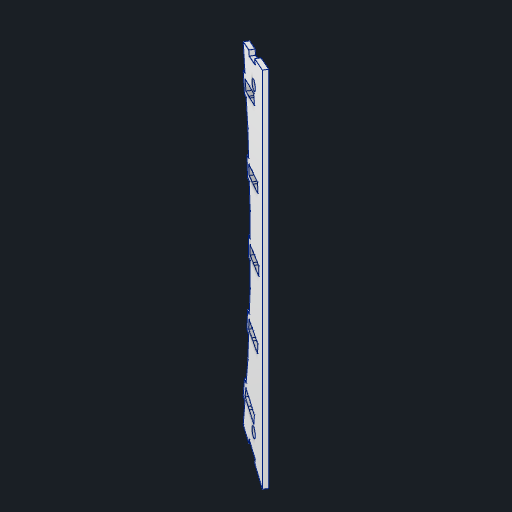
# Autodesk Inventor part: Front Plate
Saved by Autodesk Inventor 2023 (Build 270158000, 158)
## iProperties
Created: 2022-06-14
Part Number: Front Plate
Material: Aluminum 6061
Document SubType Name: Modeling
Designer: FizzyApple12
Density: 2.7 g/cm^3
Appearance: Aluminum - Flat
Author: FizzyApple12
Autodesk Inventor part; units mm, degrees
ref_plane "YZ Plane" through (0, 0, 0) normal (1, 0, 0) x (0, 1, 0)
ref_plane "XZ Plane" through (0, 0, 0) normal (0, 1, 0) x (-1, 0, 0)
ref_plane "Work Plane1" through (3.175, 0, 0) normal (0.5244795, 0, -0.8514231) x (-0.8328174, 0.2079117, -0.5130184)
sketch "Sketch1" plane through (3.175, 0, 0) normal (0.5244795, 0, -0.8514231) x (-0.8328174, 0.2079117, -0.5130184)
  line L0 (-4.273, 0.9083) -> (1.0154, -0.2158) construction
  line L1 (3.6558, 12.2067) -> (-1.6326, 13.3307) construction
  line L2 (-4.273, 0.9083) -> (-7.6513, -14.9853) projected
  line L3 (1.7457, 29.2243) -> (-1.6326, 13.3307) projected
  line L4 (6.9133, 45.2244) -> (1.8922, 29.771) projected
  line L5 (6.9133, 45.2244) -> (12.0552, 43.5536) construction
  line L6 (15.9798, 55.6321) -> (10.8378, 57.3028) construction
  line L7 (15.8589, 72.7562) -> (10.8378, 57.3028) projected
  line L8 (22.6707, 88.1284) -> (16.0618, 73.2845) projected
  line L9 (32.7754, 97.5314) -> (27.8362, 99.7304) construction
  line L10 (22.6707, 88.1284) -> (27.6098, 85.9294) construction
  line L11 (34.4452, 114.5743) -> (27.8362, 99.7304) projected
  line L12 (1.0154, -0.2158) -> (2.6442, -0.562) construction
  line L13 (2.6442, -0.562) -> (5.2847, 11.8604) construction
  line L14 (5.2847, 11.8604) -> (3.6558, 12.2067) construction
  line L15 (13.639, 43.0391) -> (17.5635, 55.1175) construction
  line L16 (12.0552, 43.5536) -> (13.639, 43.0391) construction
  line L17 (17.5635, 55.1175) -> (15.9798, 55.6321) construction
  line L18 (27.6098, 85.9294) -> (29.1311, 85.2521) construction
  line L19 (29.1311, 85.2521) -> (34.2966, 96.8541) construction
  line L20 (34.2966, 96.8541) -> (32.7754, 97.5314) construction
  line L21 (-12.4939, -90.0078) -> (-12.4939, -106.2565) projected
  line L22 (-12.4939, -90.0078) -> (-7.0873, -90.0078) construction
  line L23 (-7.0873, -90.0078) -> (-5.4221, -90.0078) construction
  line L24 (-5.4221, -90.0078) -> (-5.4221, -77.3078) construction
  line L25 (-5.4221, -77.3078) -> (-7.0873, -77.3078) construction
  line L26 (-7.0873, -77.3078) -> (-12.4939, -77.3078) construction
  line L27 (-12.4939, -61.0592) -> (-12.4939, -77.3078) projected
  line L28 (-10.7658, -44.3344) -> (-12.4643, -60.494) projected
  line L29 (-10.7658, -44.3344) -> (-5.3889, -44.8995) construction
  line L30 (-5.3889, -44.8995) -> (-3.7328, -45.0736) construction
  line L31 (-3.7328, -45.0736) -> (-2.4053, -32.4431) construction
  line L32 (-2.4053, -32.4431) -> (-4.0614, -32.2691) construction
  line L33 (-4.0614, -32.2691) -> (-9.4383, -31.7039) construction
  line L34 (-7.7398, -15.5443) -> (-9.4383, -31.7039) projected
  line L35 (-7.6513, -14.9853) -> (-7.7398, -15.5443)
  line L36 (-12.4939, -61.0592) -> (-12.4643, -60.494)
  line L37 (16.0618, 73.2845) -> (15.8589, 72.7562)
  line L38 (1.7457, 29.2243) -> (1.8922, 29.771)
  line L39 (-5.4221, -90.0078) -> (-12.4939, -90.0078)
  line L40 (-12.4939, -77.3078) -> (-5.4221, -77.3078)
  line L41 (-8.958, -90.0078) -> (-8.958, -77.3078)
  line L42 (-10.7658, -44.3344) -> (-3.7328, -45.0736)
  line L43 (-2.4053, -32.4431) -> (-9.4383, -31.7039)
  line L44 (-5.9218, -32.0735) -> (-7.2493, -44.704)
  line L45 (-4.273, 0.9083) -> (2.6442, -0.562)
  line L46 (5.2847, 11.8604) -> (-1.6326, 13.3307)
  line L47 (1.8261, 12.5956) -> (-0.8144, 0.1731)
  line L48 (6.9133, 45.2244) -> (13.639, 43.0391)
  line L49 (17.5635, 55.1175) -> (10.8378, 57.3028)
  line L50 (14.2007, 56.2101) -> (10.2761, 44.1317)
  line L51 (22.6707, 88.1284) -> (29.1311, 85.2521)
  line L52 (34.2966, 96.8541) -> (27.8362, 99.7304)
  line L53 (31.0664, 98.2923) -> (25.9009, 86.6902)
  line L54 (-12.4939, -106.2565) -> (-51.5354, -97.958)
  line L55 (-51.5354, -97.958) -> (-4.5964, 122.8728)
  line L56 (-4.5964, 122.8728) -> (34.4452, 114.5743)
  dimension "d1" = 29.21
  constraints: 44 end point, 10 midpoint, 5 parallel, 4 collinear, 1 horizontal
  measures "d1" distance between parallel lines of L47 L55
extrude "Extrusion1" add sketch "Sketch1" against normal blind 3.175
sketch "Sketch3" plane through (1.5098, 0, 2.7033) normal (-0.5244795, 0, 0.8514231) x (0.8328174, -0.2079117, 0.5130184)
  line L0 (4.5964, 122.8728) -> (-34.4452, 114.5743) projected
  line L1 (12.4939, -106.2565) -> (51.5354, -97.958) projected
  line L2 (51.5354, -97.958) -> (4.5964, 122.8728) projected
  line L3 (51.5354, -97.958) -> (53.8199, -108.7056)
  line L4 (53.8199, -108.7056) -> (37.2048, -107.8349)
  line L5 (24.5222, -107.1702) -> (12.4939, -106.5398)
  line L6 (12.4939, -90.0078) -> (12.4939, -106.2565) projected
  line L7 (12.4939, -106.5398) -> (12.4939, -106.2565)
  line L8 (-23.8284, 120.3014) -> (-34.5604, 114.8332)
  line L9 (-34.4452, 114.5743) -> (4.5964, 122.8728) projected
  line L10 (-34.5604, 114.8332) -> (-34.4452, 114.5743)
  line L11 (4.5964, 122.8728) -> (2.3119, 133.6205)
  line L12 (2.3119, 133.6205) -> (-12.5126, 126.0671)
  line L13 (-34.4452, 114.5743) -> (-27.8362, 99.7304) projected
  line L14 (-20.9994, 121.7428) -> (-15.3415, 124.6257) projected
  line L15 (-19.558, 118.9139) -> (-20.9994, 121.7428) projected
  line L16 (-13.9001, 121.7967) -> (-19.558, 118.9139) projected
  line L17 (-13.9001, 121.7967) -> (-15.3415, 124.6257) projected
  line L18 (27.859, -104.1657) -> (34.2003, -104.4981) projected
  line L19 (27.6929, -107.3364) -> (27.859, -104.1657) projected
  line L20 (34.0342, -107.6687) -> (27.6929, -107.3364) projected
  line L21 (34.0342, -107.6687) -> (34.2003, -104.4981) projected
  line L22 (24.6884, -103.9996) -> (27.859, -104.1657) projected
  line L23 (24.5222, -107.1702) -> (24.6884, -103.9996) projected
  line L24 (27.6929, -107.3364) -> (24.5222, -107.1702) projected
  line L25 (27.6929, -107.3364) -> (27.859, -104.1657) projected
  line L26 (34.2003, -104.4981) -> (37.371, -104.6642) projected
  line L27 (34.0342, -107.6687) -> (34.2003, -104.4981) projected
  line L28 (37.2048, -107.8349) -> (34.0342, -107.6687) projected
  line L29 (37.371, -104.6642) -> (37.2048, -107.8349) projected
  line L30 (-15.3415, 124.6257) -> (-12.5126, 126.0671) projected
  line L31 (-13.9001, 121.7967) -> (-15.3415, 124.6257) projected
  line L32 (-11.0712, 123.2381) -> (-13.9001, 121.7967) projected
  line L33 (-12.5126, 126.0671) -> (-11.0712, 123.2381) projected
  line L34 (-23.8284, 120.3014) -> (-20.9994, 121.7428) projected
  line L35 (-22.3869, 117.4725) -> (-23.8284, 120.3014) projected
  line L36 (-19.558, 118.9139) -> (-22.3869, 117.4725) projected
  line L37 (-19.558, 118.9139) -> (-20.9994, 121.7428) projected
  point P0 (-2.6442, -0.562)
  point P1 (-13.9001, 121.7967)
  point P2 (-19.558, 118.9139)
  point P3 (27.859, -104.1657)
  point P4 (34.2003, -104.4981)
  constraints: 16 end point, 4 collinear, 4 parallel
extrude "Extrusion2" add sketch "Sketch3" against normal blind 3.175 contours L0 L10 L8 L35 L36 L16 L32 L33 L12 L11 | L1 L3 L4 L29 L26 L18 L22 L23 L5 L7
sketch "Sketch4" plane through (1.5098, 0, 2.7033) normal (-0.5244795, 0, 0.8514231) x (0.8328174, -0.2079117, 0.5130184)
  line L0 (31.0297, -104.3319) -> (31.6943, -91.6493) construction
  line L1 (-16.7291, 120.3553) -> (-10.9634, 109.0395) construction
  line L2 (31.6943, -91.6493) -> (-10.9634, 109.0395) construction
  line L3 (24.6884, -103.9996) -> (37.371, -104.6642) construction
  line L4 (-11.0712, 123.2381) -> (-22.3869, 117.4725) construction
  point P0 (-2.6442, -0.562)
  point P1 (10.3655, 8.6951)
  dimension "d17" = 12.7
  dimension "d18" = 12.7
  constraints: 6 end point, 3 midpoint, 2 coincident, 2 perpendicular
  measures "d17" distance of L0.start L0.end
  measures "d18" distance of L1.start L1.end
hole "Hole2" at (11.6816, -96.2362, 8.9691) at (11.6815, 108.9362, 8.9691) at (11.6816, 6.35, 8.9691) direction (0.5244795, 0, -0.8514231) diameter 6.7564 depth 13.6144 clearance for "Flat Head Machine Screw (82)" size "1/4" standard "Ansi Unified Screw Threads"
sketch "Sketch5" plane through (3.175, 0, 0) normal (0.5244795, 0, -0.8514231) x (-0.8328174, 0.2079117, -0.5130184)
  line L0 (1.8261, 12.5956) -> (-0.8144, 0.1731) construction
  line L1 (0.5058, 6.3843) -> (-11.9167, 9.0248) construction
  line L2 (-0.8144, 0.1731) -> (1.8261, 12.5956) projected
  line L3 (-21.5406, 7.8245) -> (-3.6129, 4.0139)
  line L4 (-3.6129, 4.0139) -> (-2.2927, 10.2251)
  line L5 (-2.2927, 10.2251) -> (-20.2204, 14.0358)
  line L6 (-20.2204, 14.0358) -> (-21.5406, 7.8245)
  line L7 (-21.5406, 7.8245) -> (-2.2927, 10.2251) construction
  line L8 (-3.6129, 4.0139) -> (-20.2204, 14.0358) construction
  line L9 (-1.6326, 13.3307) -> (1.7457, 29.2243) projected
  line L10 (10.2761, 44.1317) -> (14.2007, 56.2101) construction
  line L11 (25.9009, 86.6902) -> (31.0664, 98.2923) construction
  line L12 (-7.2493, -44.704) -> (-5.9218, -32.0735) construction
  line L13 (-8.958, -90.0078) -> (-8.958, -77.3078) construction
  line L14 (-6.5855, -38.3887) -> (-19.216, -37.0612) construction
  line L15 (-8.958, -77.3078) -> (-8.958, -90.0078) construction
  line L16 (-8.958, -83.6578) -> (-21.658, -83.6578) construction
  line L17 (28.4836, 92.4912) -> (16.8816, 97.6568) construction
  line L18 (12.2384, 50.1709) -> (0.16, 54.0954) construction
  line L19 (-28.6618, -39.2609) -> (-10.4339, -41.1768)
  line L20 (-10.4339, -41.1768) -> (-9.7702, -34.8615)
  line L21 (-9.7702, -34.8615) -> (-27.998, -32.9457)
  line L22 (-27.998, -32.9457) -> (-28.6618, -39.2609)
  line L23 (-28.6618, -39.2609) -> (-9.7702, -34.8615) construction
  line L24 (-10.4339, -41.1768) -> (-27.998, -32.9457) construction
  line L25 (-30.8221, -86.8328) -> (-12.4939, -86.8328)
  line L26 (-12.4939, -86.8328) -> (-12.4939, -80.4828)
  line L27 (-12.4939, -80.4828) -> (-30.8221, -80.4828)
  line L28 (-30.8221, -80.4828) -> (-30.8221, -86.8328)
  line L29 (-30.8221, -86.8328) -> (-12.4939, -80.4828) construction
  line L30 (-12.4939, -86.8328) -> (-30.8221, -80.4828) construction
  line L31 (-9.5367, 53.9077) -> (7.8944, 48.244)
  line L32 (7.8944, 48.244) -> (9.8567, 54.2832)
  line L33 (9.8567, 54.2832) -> (-7.5745, 59.9469)
  line L34 (-7.5745, 59.9469) -> (-9.5367, 53.9077)
  line L35 (-9.5367, 53.9077) -> (9.8567, 54.2832) construction
  line L36 (7.8944, 48.244) -> (-7.5745, 59.9469) construction
  line L37 (7.2184, 98.4837) -> (23.9621, 91.0289)
  line L38 (23.9621, 91.0289) -> (26.5448, 96.8299)
  line L39 (26.5448, 96.8299) -> (9.8012, 104.2847)
  line L40 (9.8012, 104.2847) -> (7.2184, 98.4837)
  line L41 (7.2184, 98.4837) -> (26.5448, 96.8299) construction
  line L42 (23.9621, 91.0289) -> (9.8012, 104.2847) construction
  point P0 (2.6442, -0.562)
  point P1 (-11.9167, 9.0248)
  dimension "d26" = 12.7
  dimension "d27" = 18.3282
  dimension "d28" = 6.35
  dimension "d29" = 9.1641
  dimension "d30" = 12.7
  dimension "d31" = 12.7
  dimension "d32" = 12.7
  dimension "d33" = 12.7
  dimension "d34" = 6.35
  dimension "d35" = 18.3282
  dimension "d36" = 6.35
  dimension "d37" = 18.3282
  dimension "d38" = 6.35
  dimension "d39" = 18.3282
  dimension "d40" = 6.35
  dimension "d41" = 18.3282
  constraints: 70 end point, 16 midpoint, 15 perpendicular, 10 parallel
  measures "d26" distance of L1.start L1.end
  measures "d27" distance of L3.start L3.end
  measures "d28" distance of L4.end L3.end
  measures "d29" distance from line of L9 point (-11.917, 9.025)
  measures "d30" distance of L14.start L14.end
  measures "d31" distance of L16.start L16.end
  measures "d32" distance of L17.start L17.end
  measures "d33" distance of L18.start L18.end
  measures "d34" distance of L20.end L19.end
  measures "d35" distance between parallel lines of L20 L22
  measures "d36" distance of L26.end L25.end
  measures "d37" distance between parallel lines of L28 L26
  measures "d38" distance of L32.end L31.end
  measures "d39" distance between parallel lines of L34 L32
  measures "d40" distance of L38.end L37.end
  measures "d41" distance between parallel lines of L38 L40
extrude "Extrusion3" cut sketch "Sketch5" against normal through all
sketch "Sketch6" plane through (1.5098, 0, 2.7033) normal (-0.5244795, 0, 0.8514231) x (0.8328174, -0.2079117, 0.5130184)
  arc A0 (9.8969, 5.3496) -> (12.1543, 5.8294) centre (10.3655, 8.6951) ccw construction
  line L0 (-1.8261, 12.5956) -> (0.8144, 0.1731) construction
  line L1 (8.958, -90.0078) -> (8.958, -77.3078) construction
  line L2 (8.958, -83.6578) -> (20.0722, -83.6578) construction
  line L3 (-25.9009, 86.6902) -> (-31.0664, 98.2923) construction
  line L4 (-28.4836, 92.4912) -> (-18.3303, 97.0118) construction
  line L5 (-10.2761, 44.1317) -> (-14.2007, 56.2101) construction
  line L6 (-12.2384, 50.1709) -> (-1.6682, 53.6054) construction
  line L7 (-14.2007, 56.2101) -> (-10.2761, 44.1317) construction
  line L8 (7.2493, -44.704) -> (5.9218, -32.0735) construction
  line L9 (6.5855, -38.3887) -> (17.6388, -37.227) construction
  line L10 (5.9218, -32.0735) -> (7.2493, -44.704) construction
  point P0 (-2.6442, -0.562)
  dimension "d44" = 11.1142
  dimension "d45" = 11.1142
  dimension "d46" = 11.1142
  dimension "d47" = 11.1142
  dimension "d48" = 11.1142
  constraints: 8 end point, 4 coincident, 4 midpoint, 3 perpendicular, 1 horizontal
  measures "d44" distance from line of A0.centre L0
  measures "d45" distance from line of L2.end L1
  measures "d46" distance of L4.start L4.end
  measures "d47" distance of L6.start L6.end
  measures "d48" distance of L9.start L9.end
hole "Hole3" at (9.6098, -40.0808, 7.6929) at (3.4171, -86.0029, 3.8782) at (9.6098, 52.7808, 7.6929) at (3.4171, 98.7029, 3.8782) direction (0.5244795, 0, -0.8514231) diameter 6.7564 depth 13.6144 clearance for "Flat Head Machine Screw (82)" size "1/4" standard "Ansi Unified Screw Threads"
equation "\"d27\" = 2 * d29"
equation "\"d34\" = d28"
equation "\"d35\" = d27"
equation "\"d36\" = d28"
equation "\"d37\" = d27"
equation "\"d38\" = d28"
equation "\"d39\" = d27"
equation "\"d40\" = d28"
equation "\"d41\" = d27"
equation "\"d45\" = d44"
equation "\"d46\" = d44"
equation "\"d47\" = d44"
equation "\"d48\" = d44"
body "Solid1"
